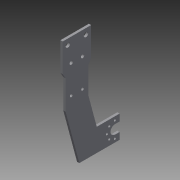
# Autodesk Inventor part: Arm_MiniLink_1
Saved by Autodesk Inventor 2013 (Build 170138000, 138)
## iProperties
Created: 2014-05-16
Part Number: Arm_MiniLink_1
Material: 一般
Document SubType Name: Modeling
Designer: andou
Density: 1 g/cm^3
Mass: 4.80785 g
Surface Area: 55.525 cm^2
Volume: 4.80785 cm^3
Author: andou
Autodesk Inventor part; units mm, degrees
ref_plane "YZ Plane" through (0, 0, 0) normal (1, 0, 0) x (0, 1, 0)
ref_plane "XZ Plane" through (0, 0, 0) normal (0, 1, 0) x (-1, 0, 0)
ref_plane "XY Plane" through (0, 0, 0) normal (0, 0, 1) x (1, 0, 0)
sketch "スケッチ1" plane through (0, 0, 0) normal (1, 0, 0) x (0, 1, 0)
  line L0 (25, 50) -> (-25, 50)
  line L1 (-25, 50) -> (-25, -50)
  line L2 (-25, -50) -> (25, -50)
  line L3 (25, -50) -> (25, 50)
  point P0 (0, 0)
  dimension "d0" = 50
  dimension "d2" = 100
  dimension "d3" = 50
  dimension "d4" = 25
  constraints: 8 end point, 2 parallel, 1 horizontal, 1 perpendicular
  measures "d0" distance of L1.end L2.end
  measures "d2" distance of L0.end L1.end
  measures "d3" distance from line of point (0, 0) L0
  measures "d4" distance from line of L1 point (0, 0)
extrude "押し出し1" add sketch "スケッチ1" along normal blind 2
sketch "スケッチ2" plane through (2, 0, 0) normal (1, 0, 0) x (0, 0, -1)
  line L0 (-50, 25) -> (-50, -25) projected
  line L1 (-50, -25) -> (50, -25) projected
  line L2 (50, -25) -> (50, 25) projected
  line L3 (50, 25) -> (-50, 25) projected
  line L4 (-25, -25) -> (-20.6699, -22.5)
  line L5 (-20.6699, -22.5) -> (4.8301, -22.5)
  line L6 (4.8301, -22.5) -> (50, -10.3968)
  line L7 (-50, 0) -> (-25, 0)
  line L8 (-25, 0) -> (-20.6699, -2.5)
  line L9 (-20.6699, -2.5) -> (2.1971, -2.5)
  line L10 (2.1971, -2.5) -> (30, 4.9498)
  line L11 (30, 4.9498) -> (30, 25)
  line L12 (-25, -25) -> (-50, -25)
  line L13 (-50, -25) -> (-50, 0)
  point P0 (0, 0)
  dimension "d7" = 150
  dimension "d8" = 150
  dimension "d9" = 25
  dimension "d10" = 25
  dimension "d11" = 25
  dimension "d12" = 20
  dimension "d13" = 2.5
  dimension "d14" = 25.5
  dimension "d16" = 165
  dimension "d17" = 20
  dimension "d18" = 20
  constraints: 20 end point, 4 parallel, 3 point on line, 2 collinear, 1 midpoint, 1 perpendicular
  measures "d7" angle of L1 L4
  measures "d8" angle of L8 L9
  measures "d9" distance of L4.start L0.end
  measures "d10" distance of L7.start L7.end
  measures "d11" distance between parallel lines of L1 L7
  measures "d12" distance between parallel lines of L5 L9
  measures "d13" distance between parallel lines of L1 L5
  measures "d14" distance of L4.end L5.end
  measures "d16" angle of L6 L5
  measures "d17" distance between parallel lines of L2 L11
  measures "d18" distance between parallel lines of L6 L10
extrude "押し出し2" cut sketch "スケッチ2" against normal blind 2 contours L7 L8 L9 L10 L11 L3 L2 L6 L5 L4 L1 L0 keep common part
sketch "スケッチ3" plane through (2, 0, 0) normal (1, 0, 0) x (0, 0, -1)
  line L0 (30, 4.9498) -> (30, 25) projected
  line L1 (2.1971, -2.5) -> (30, 4.9498) projected
  line L2 (-20.6699, -2.5) -> (2.1971, -2.5) projected
  line L3 (-25, 0) -> (-20.6699, -2.5) projected
  line L4 (-50, 0) -> (-25, 0) projected
  line L5 (-50, 0) -> (-50, -25) projected
  line L6 (-50, -25) -> (-25, -25) projected
  line L7 (-20.6699, -22.5) -> (-25, -25) projected
  line L8 (4.8301, -22.5) -> (-20.6699, -22.5) projected
  line L9 (50, -10.3968) -> (4.8301, -22.5) projected
  line L10 (50, -10.3968) -> (50, 25) projected
  line L11 (50, 25) -> (30, 25) projected
  circle A0 centre (-45, -4.5) radius 2
  circle A1 centre (-45, -20.5) radius 2
  circle A2 centre (-30, -7.5) radius 1.5
  circle A3 centre (-30, -17.5) radius 1.5
  arc A4 (36, 21) -> (44, 21) centre (40, 21) ccw
  line L12 (36, 21) -> (36, 25)
  line L13 (44, 21) -> (44, 25)
  point P0 (0, 0)
  dimension "d21" = 8
  dimension "d25" = 4
  dimension "d30" = 6
  dimension "d31" = 4
  dimension "d35" = 10
  dimension "d36" = 16
  dimension "d37" = 7.5
  dimension "d38" = 4.5
  dimension "d40" = 5
  dimension "d41" = 5
  dimension "d61" = 3
  dimension "d68" = 15
  dimension "d69" = 15
  constraints: 5 centre point, 4 end point, 2 equal radius, 2 perpendicular, 2 point on circle, 2 point on line, 2 tangent
  measures "d21" diameter of A4
  measures "d25" diameter of A0
  measures "d30" distance between parallel lines of L0 L12
  measures "d31" distance from line of L11 A4.centre
  measures "d35" distance of A3.centre A2.centre
  measures "d36" distance of A0.centre A1.centre
  measures "d37" distance from line of A3.centre L6
  measures "d38" distance from line of L6 A1.centre
  measures "d40" distance from line of A1.centre L5
  measures "d41" distance from line of L5 A0.centre
  measures "d61" diameter of A2
  measures "d68" horizontal distance of A0.centre A2.centre
  measures "d69" horizontal distance of A3.centre A1.centre
extrude "押し出し5" cut sketch "スケッチ3" against normal blind 2 contours L0 L11 L12 A4 L13 L10 L9 L8 L7 L6 L5 L4 L3 L2 L1 keep common part
sketch "スケッチ4" plane through (2, 0, 0) normal (1, 0, 0) x (0, 0, -1)
  line L0 (50, 25) -> (30, 25) projected
  circle A0 centre (33, 21) radius 1
  arc A1 (36, 21) -> (44, 21) centre (40, 21) ccw projected
  point P0 (0, 0)
  dimension "d47" = 4
  dimension "d49" = 2
  dimension "d64" = 7
  constraints: 1 centre point
  measures "d47" distance from line of L0 A0.centre
  measures "d49" diameter of A0
  measures "d64" distance of A1.centre A0.centre
hole "穴1" at (2, 21, -33) direction (-1, 0, 0) diameter 2 end through all
pattern_circular "円形状パターン2" count 5 over 180 about axis through (2, 21, -40) along (1, 0, 0) of "穴1"
sketch "スケッチ5" plane through (2, 0, 0) normal (1, 0, 0) x (0, 0, -1)
  line L0 (-20.6699, -2.5) -> (2.1971, -2.5) projected
  circle A0 centre (-30, -7.5) radius 1.5 projected
  circle A1 centre (-30, -17.5) radius 1.5 projected
  circle A2 centre (-5, -7.5) radius 1
  circle A3 centre (-5, -17.5) radius 1
  point P0 (0, 0)
  dimension "d70" = 2
  dimension "d74" = 5
  dimension "d75" = 10
  dimension "d76" = 25
  dimension "d77" = 25
  constraints: 2 centre point, 1 equal radius
  measures "d70" diameter of A3
  measures "d74" distance from line of L0 A2.centre
  measures "d75" distance of A2.centre A3.centre
  measures "d76" distance of A1.centre A3.centre
  measures "d77" distance of A0.centre A2.centre
hole "穴2" at (2, -7.5, 5) at (2, -17.5, 5) direction (-1, 0, 0) diameter 2.5 end through all
